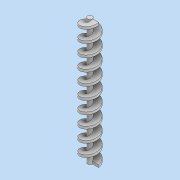
# Autodesk Inventor part: spiral shaft
Saved by Autodesk Inventor 2020 (Build 240168000, 168)
## iProperties
Created: 2020-12-17
Part Number: spiral shaft
Material: Generic
Document SubType Name: Modeling
Designer: solar
Density: 1 g/cm^3
Appearance: Default
Author: solar
Autodesk Inventor part; units mm, degrees
ref_plane "YZ Plane" through (0, 0, 0) normal (1, 0, 0) x (0, 1, 0)
ref_plane "XZ Plane" through (0, 0, 0) normal (0, 1, 0) x (-1, 0, 0)
ref_plane "XY Plane" through (0, 0, 0) normal (0, 0, 1) x (1, 0, 0)
sketch "Sketch1" plane through (0, 0, 0) normal (0, 0, 1) x (1, 0, 0)
  line L0 (0, 0) -> (10, 0)
  line L1 (10, 0) -> (10, -5)
  line L2 (10, 0) -> (10, 5)
  line L3 (10, 5) -> (35, 5)
  line L4 (35, 5) -> (35, -5)
  line L5 (35, -5) -> (10, -5)
  dimension "d2" = 10
  dimension "d3" = 5
  dimension "d4" = 5
  dimension "d5" = 25
  dimension "d6" = 10
  constraints: 12 end point, 3 perpendicular, 1 horizontal, 1 vertical
  measures "d2" distance of L0.start L0.end
  measures "d3" distance of L0.end L1.end
  measures "d4" distance of L0.end L2.end
  measures "d5" distance of L2.end L3.end
  measures "d6" distance of L3.end L4.end
coil "Coil1" sketch "Sketch1" operation add axis through (0, -10, 0) along (0, -1, 0) pitch 50 turns 10 hand right
sketch "Sketch2" plane through (0, 0, 0) normal (0, 1, 0) x (-1, 0, 0)
  circle A0 centre (0, 0) radius 10
  point P0 (-10, 0)
  constraints: 1 coincident, 1 horizontal alignment, 2 other
extrude "Extrusion1" add sketch "Sketch2" along normal blind 5
extrude "Extrusion2" add sketch "Sketch2" against normal blind 505
body "Solid1"
